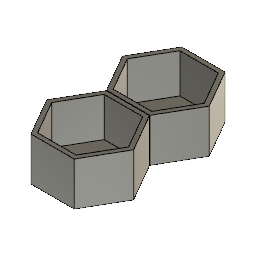
parts holder v1 (Autodesk Fusion 360 design; units mm, degrees)
Autodesk Fusion 360 part; units mm, degrees
sketch "base" plane through (0, 0, 0) normal (0, 0, 1) x (1, 0, 0)
  line L0 (-12.7, 21.997) -> (-25.4, 0)
  line L1 (-25.4, 0) -> (-12.7, -21.997)
  line L2 (-12.7, -21.997) -> (12.7, -21.997)
  line L3 (12.7, -21.997) -> (25.4, 0)
  line L4 (25.4, 0) -> (12.7, 21.997)
  line L5 (12.7, 21.997) -> (-12.7, 21.997)
  line L6 (25.4, 44.196) -> (12.7, 66.193)
  line L7 (12.7, 66.193) -> (-12.7, 66.193)
  line L8 (12.7, 22.199) -> (25.4, 44.196)
  line L9 (-12.7, 22.199) -> (12.7, 22.199)
  line L10 (-12.7, 66.193) -> (-25.4, 44.196)
  line L11 (-25.4, 44.196) -> (-12.7, 22.199)
  point P0 (0, 44.196)
  dimension "d1" = 25.4
  dimension "d2" = 25.4
  dimension "d3" = 44.196
  constraint horizontal L2
  constraint horizontal L9
  measures "d1" distance of L1.end L2.end
  measures "d2" distance of L9.start L8.start
  measures "d3" distance of L3.end L6.start
extrude "Extrude1" add sketch "base" along normal blind 25.4 makes body 1 at (-4.2333, -7.3323, 0) makes body 2 at (-8.4667, 44.196, 0)
shell "Shell1" thickness 2.54 removed faces 1 at (-4.2333, -7.3323, 25.4) on bodies 1
shell "Shell2" thickness 2.54 removed faces 1 at (-8.4667, 44.196, 25.4) on bodies 2
